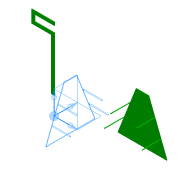
# Autodesk Inventor part: PyramidMockup
Saved by Autodesk Inventor 2012 (Build 160160000, 160)
## iProperties
Created: 2013-01-12
Part Number: PyramidMockup
Material: Default
Document SubType Name: Modeling
Designer: JesseK
Surface Area: 92934.9 cm^2
Volume: 110620 cm^3
Author: JesseK
Autodesk Inventor part; units mm, degrees
ref_plane "YZ Plane" through (0, 0, 0) normal (1, 0, 0) x (0, 1, 0)
ref_plane "XZ Plane" through (0, 0, 0) normal (0, 1, 0) x (-1, 0, 0)
ref_plane "XY Plane" through (0, 0, 0) normal (0, 0, 1) x (1, 0, 0)
sketch "Sketch1" plane through (0, 0, 0) normal (0, 0, 1) x (1, 0, 0)
  line L0 (0, 0) -> (2387.6, 0)
  line L1 (2387.6, 0) -> (1498.6, 2286)
  line L2 (1498.6, 2286) -> (889, 2286)
  line L3 (889, 2286) -> (0, 0)
  dimension "d0" = 609.6
  dimension "d1" = 2387.6
  dimension "d2" = 2286
  constraints: 8 end point, 2 horizontal, 1 equal length
  measures "d0" distance of L1.end L2.end
  measures "d1" distance of L0.start L0.end
  measures "d2" distance between parallel lines of L0 L2
extrude "Extrusion1" add sketch "Sketch1" along normal blind 25.4
sketch "Sketch2" plane through (0, 0, 25.4) normal (0, 0, 1) x (1, 0, 0)
  line L0 (0, 0) -> (889, 2286) projected
  circle A0 centre (572.2269, 1524) radius 19.05
  circle A1 centre (275.8935, 762) radius 19.05
  line L1 (1498.6, 2286) -> (2387.6, 0) projected
  circle A2 centre (1815.3731, 1524) radius 19.05
  circle A3 centre (2111.7065, 762) radius 19.05
  line L2 (572.2269, 1524) -> (1815.3731, 1524) construction
  line L3 (275.8935, 762) -> (2111.7065, 762) construction
  dimension "d5" = 38.1
  dimension "d6" = 762
  dimension "d7" = 1524
  constraints: 4 centre point, 4 end point, 4 tangent, 3 equal radius, 2 horizontal
  measures "d5" diameter of A0
  measures "d6" vertical distance of L0.start L3.start
  measures "d7" vertical distance of L0.start L2.start
extrude "Extrusion2" add sketch "Sketch2" along normal blind 914.4
sketch "Sketch3" plane through (0, 0, 25.4) normal (0, 0, 1) x (1, 0, 0)
  line L0 (0, 0) -> (293.6482, 755.0954) projected
  line L1 (2387.6, 0) -> (0, 0) projected
  line L2 (0, 0) -> (0.7819, 2.0105)
  line L3 (0.7819, 0) -> (0.7819, 2.0105)
  line L4 (0.7819, 0) -> (0, 0)
  line L5 (0.7819, 0) -> (9.8778, 25.4)
  line L6 (9.8778, 25.4) -> (9.8778, 0)
  line L7 (9.8778, 0) -> (0.7819, 0)
  dimension "d10" = 25.4
  constraints: 12 end point, 4 point on line, 2 horizontal, 2 vertical
  measures "d10" distance of L5.end L6.end
extrude "Extrusion3" cut sketch "Sketch3" against normal through all contours L5 L6 L1
sketch "Sketch4" plane through (0, 0, 25.4) normal (0, 0, 1) x (1, 0, 0)
  line L0 (-3241.3222, 0) -> (-3241.3222, 2492.375)
  line L1 (-3241.3222, 2492.375) -> (-4201.0707, 2492.375)
  line L2 (-4201.0707, 2492.375) -> (-4201.0707, 3101.975)
  line L3 (-4201.0707, 3101.975) -> (-3088.9222, 3101.975)
  line L4 (-3088.9222, 3101.975) -> (-3088.9222, 2949.575)
  line L5 (-3088.9222, 2949.575) -> (-4048.6707, 2949.575)
  line L6 (-4048.6707, 2949.575) -> (-4048.6707, 2644.775)
  line L7 (-4048.6707, 2644.775) -> (-3088.9222, 2644.775)
  line L8 (-3088.9222, 2644.775) -> (-3088.9222, 0)
  line L9 (-3088.9222, 0) -> (-3241.3222, 0)
  line L10 (-3088.9222, 0) -> (0, 0) construction
  point P0 (9.8778, 0)
  dimension "d13" = 152.4
  dimension "d14" = 152.4
  dimension "d15" = 152.4
  dimension "d16" = 304.8
  dimension "d17" = 2644.775
  dimension "d18" = 3098.8
  constraints: 22 end point, 6 horizontal, 5 vertical, 1 coincident, 1 collinear, 1 parallel
  measures "d13" distance between parallel lines of L8 L0
  measures "d14" distance between parallel lines of L7 L1
  measures "d15" distance between parallel lines of L3 L5
  measures "d16" distance of L5.end L6.end
  measures "d17" distance between parallel lines of L9 L7
  measures "d18" distance of point (9.878, 0) L8.end
extrude "Extrusion4" add sketch "Sketch4" against normal blind 25.4
body "Solid1"
